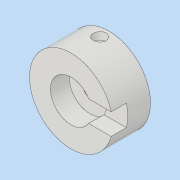
# Autodesk Inventor part: EncoderDisc
Saved by Autodesk Inventor 2017 (Build 210142000, 142)
## iProperties
Created: 2017-11-01
Part Number: EncoderDisc
Material: ABS Plastic
Document SubType Name: Modeling
Designer: Derek Wider
Density: 1.06 g/cm^3
Appearance: Smooth - White
Author: Derek Wider
Autodesk Inventor part; units mm, degrees
ref_plane "YZ Plane" through (0, 0, 0) normal (1, 0, 0) x (0, 1, 0)
ref_plane "XY Plane" through (0, 0, 0) normal (0, 0, 1) x (1, 0, 0)
sketch "Sketch1" plane through (0, 0, 0) normal (0, 0, 1) x (1, 0, 0)
  circle A0 centre (0, 0) radius 11.1125
  circle A1 centre (0, 0) radius 5.5245
  circle A2 centre (0, 0) radius 1.8415
  dimension "d0" = 22.225
  dimension "d1" = 11.049
  dimension "d2" = 3.683
  constraints: 3 centre point, 3 coincident
  measures "d0" diameter of A0
  measures "d1" diameter of A1
  measures "d2" diameter of A2
extrude "Extrusion1" add sketch "Sketch1" along normal blind 10.16 contours A0
extrude "Extrusion2" add sketch "Sketch1" along normal blind 5.08 contours A1
sketch "Sketch2" plane through (0, 0, 0) normal (1, 0, 0) x (0, 1, 0)
  line L0 (11.1125, 10.16) -> (-11.1125, 10.16) projected
  line L1 (2.8575, 10.16) -> (-2.8575, 10.16)
  line L2 (-2.8575, 10.16) -> (-2.8575, 6.096)
  line L3 (-2.8575, 6.096) -> (2.8575, 6.096)
  line L4 (2.8575, 6.096) -> (2.8575, 10.16)
  point P0 (0, 0)
  dimension "d7" = 5.715
  dimension "d8" = 2.8575
  dimension "d9" = 4.064
  constraints: 8 end point, 2 parallel, 1 horizontal, 1 perpendicular, 1 point on line
  measures "d7" distance between parallel lines of L2 L4
  measures "d8" distance from line of point (0, 0) L2
  measures "d9" distance of L3.end L1.start
extrude "Extrusion3" cut sketch "Sketch2" along normal through all
ref_plane "Work Plane1" through (0, 11.1125, 0) normal (0, 1, 0) x (-1, 0, 0)
sketch "Sketch3" plane through (0, 11.1125, 0) normal (0, 1, 0) x (-1, 0, 0)
  line L0 (11.1125, 0) -> (11.1125, 10.16) construction
  circle A0 centre (0, 2.54) radius 1.7145
  point P0 (0, 0)
  dimension "d12" = 3.429
  dimension "d13" = 2.54
  constraints: 1 centre point
  measures "d12" diameter of A0
  measures "d13" distance of point (0, 0) A0.centre
extrude "Extrusion4" cut sketch "Sketch3" against normal blind 2.032
equation "\"d5\" = 0.5 * d3"
equation "\"d8\" = 0.5 * d7"
equation "\"d10\" = 0.5 * d3"
equation "\"d3\" = 10.16"
body "Solid1"
